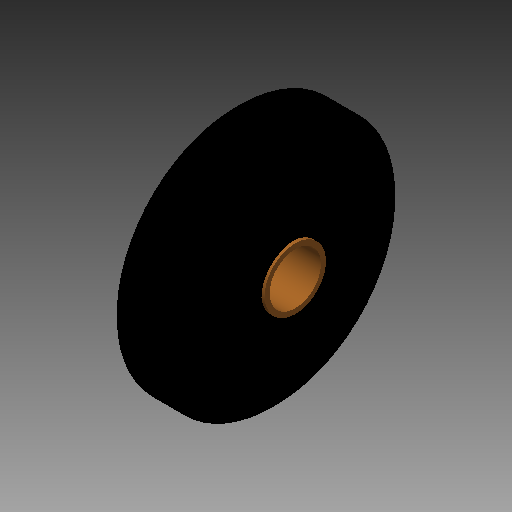
# Autodesk Inventor part: 2281_w
Saved by Autodesk Inventor 2019 (Build 230136000, 136)
## iProperties
Category: PARTsolutions
Company: 8020
Created: 2019-11-08
Part Number: 2281_w
Material: Generic
Catalog Web Link: www.cadenas.de
Description: 2281, 2282, 2280, 2290_w-Roller Wheels
Vendor: 8020
Document SubType Name: Modeling
Designer: psadmin
Manufacturer: 8020
Mass: 10.2129 g
Surface Area: 36.2018 cm^2
Volume: 10.2129 cm^3
Density: 1 g/cm^3
Appearance: PSOLRGB-192-192-192
PSOL_IDENT_0: {$CADENAS_DATA\23d-libs\8020\inch\linear_motion\2281.prj},175 {VTYP=3D},{NB=2281_w},{LINA=2281_w},{N
PSOL_IDENT_1: N=2281, 2282, 2280, 2290_w},{DATE=01.10.2019 06:04:24},{GEOMDATE=01.03.2012 00:00:00},{VERSION=},{LI
PSOL_IDENT_2: NEID=10},{WBVAR=BT,RI},{WBNUMERIC=}  {NB=2281_w},{LINA=2281_w},{KT=DUMMY},{PN=2281},{NO=1},{MAT=Self
PSOL_IDENT_3: -lubricating, fiberglass-reinforced black nylon.},{BT=2},{BT1= '2','Permanent Lubricated Bronze Bush
PSOL_IDENT_4: ing' },{MT=10 Series},{RI=10},{RI1= '10','10 Series','15','15 Series' },{A=1.500},{B=1.125},{C=0.240
PSOL_IDENT_5: },{D=0.480},{E=0.563},{F=0.188},{G=0.314},{H=0.214},{J=0.118},{K=0.622},{L=0.429},{M=0.320},{N=1/4-2
PSOL_IDENT_6: 0},{N1=0.2500},{P=0.060},{Q=0.378},{W=.070},{G1=0.375},{K1=0.000},{NTP=3382}
NN: 2281, 2282, 2280, 2290_w
NT: Roller Wheels
NB: 2281_w
NBSYN: $PN._w
LINA: 2281_w
PN: 2281
MAT: Self-lubricating, fiberglass-reinforced black nylon.
BT: Permanent Lubricated Bronze Bushing
MT: 10 Series
RI: 10 Series
A: 1.5
B: 1.125
C: 0.24
D: 0.48
E: 0.563
F: 0.188
G: 0.314
H: 0.214
J: 0.118
K: 0.622
L: 0.429
M: 0.32
N: 1/4-20
P: 0.06
Q: 0.378
W: .070
NTP: 3382
SUPPLIER: 8020
ARTICLENO: 2281_w
BOMINFO: 2281_w
CREATOR: CADENAS GmbH
Title: 2281_w
Author: Cadenas PARTsolutions
Comments: Roller Wheels
Autodesk Inventor part; units mm, degrees
sketch "Sketch_1" plane through (0, 0, 0) normal (0, 0, 1) x (1, 0, 0)
  line L0 (6.096, 0) -> (-6.096, 0)
  line L1 (-6.096, 5.2705) -> (-5.588, 4.7625)
  line L2 (-5.588, 4.7625) -> (5.588, 4.7625)
  line L3 (5.588, 4.7625) -> (6.096, 5.2705)
  line L4 (6.096, 5.2705) -> (6.096, 13.7795)
  line L5 (6.096, 13.7795) -> (5.588, 14.2875)
  line L6 (5.588, 14.2875) -> (3.8354, 14.2875)
  arc A0 (3.048, 15.0749) -> (3.8354, 14.2875) centre (3.8354, 15.0749) ccw
  line L7 (3.048, 15.0749) -> (3.048, 18.542)
  line L8 (3.048, 18.542) -> (2.54, 19.05)
  line L9 (2.54, 19.05) -> (-2.54, 19.05)
  line L10 (-2.54, 19.05) -> (-3.048, 18.542)
  line L11 (-3.048, 18.542) -> (-3.048, 15.0749)
  arc A1 (-3.8354, 14.2875) -> (-3.048, 15.0749) centre (-3.8354, 15.0749) ccw
  line L12 (-3.8354, 14.2875) -> (-5.588, 14.2875)
  line L13 (-5.588, 14.2875) -> (-6.096, 13.7795)
  line L14 (-6.096, 13.7795) -> (-6.096, 5.2705)
  constraints: 30 end point, 4 point on circle, 2 centre point
revolve "Revolution1" add sketch "Sketch_1" angle 360 about axis through (6.096, 0, 0) along (1, 0, 0)
sketch "Sketch_2" plane through (0, 0, 0) normal (0, 0, 1) x (1, 0, 0)
  line L0 (6.096, 0) -> (-6.096, 0)
  line L1 (-6.096, 4.7625) -> (-6.096, 3.9878)
  line L2 (-6.096, 3.9878) -> (6.096, 3.9878)
  line L3 (6.096, 3.9878) -> (6.096, 4.7625)
  line L4 (6.096, 4.7625) -> (-6.096, 4.7625)
  constraints: 10 end point
revolve "Revolution2" add sketch "Sketch_2" angle 360 about axis through (6.096, 0, 0) along (1, 0, 0)
ref_plane "to_bolt_XY" through (6.096, 0, 0) normal (1, 0, 0) x (0, 0, -1)
ref_plane "to_bolt_YZ" through (6.096, 0, 0) normal (0, 0, -1) x (0, 1, 0)
ref_plane "to_bolt_ZX" through (6.096, 0, 0) normal (0, 1, 0) x (1, 0, 0)
ref_plane "wheel_XY" through (0, 0, 0) normal (1, 0, 0) x (0, 0, -1)
ref_plane "wheel_YZ" through (0, 0, 0) normal (0, 0, -1) x (0, 1, 0)
ref_plane "wheel_ZX" through (0, 0, 0) normal (0, 1, 0) x (1, 0, 0)
body "Solid1"
